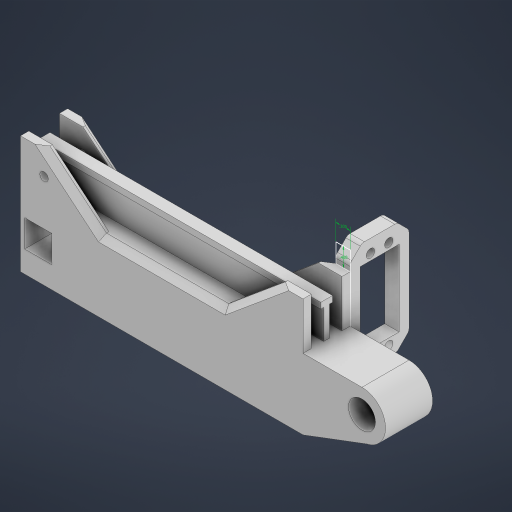
# Autodesk Inventor part: Drone_Launcher_Base2
Saved by Autodesk Inventor 2023 (Build 270158000, 158)
## iProperties
Created: 2024-02-18
Part Number: Drone_Launcher_Base2
Material: Generic
Document SubType Name: Modeling
Designer: kelle
Density: 1 g/cm^3
Appearance: Default
Author: kelle
Autodesk Inventor part; units mm, degrees
ref_plane "YZ Plane" through (0, 0, 0) normal (1, 0, 0) x (0, 1, 0)
ref_plane "XZ Plane" through (0, 0, 0) normal (0, 1, 0) x (-1, 0, 0)
ref_plane "XY Plane" through (0, 0, 0) normal (0, 0, 1) x (1, 0, 0)
sketch "Sketch1" plane through (0, 0, 0) normal (0, 0, 1) x (1, 0, 0)
  line L0 (76.2, -19.05) -> (-76.2, -19.05)
  line L1 (-76.2, -19.05) -> (-76.2, 19.05)
  line L2 (-76.2, 19.05) -> (76.2, 19.05)
  line L3 (76.2, 19.05) -> (76.2, -19.05)
  line L4 (76.2, -19.05) -> (-76.2, 19.05) construction
  line L5 (-76.2, -19.05) -> (76.2, 19.05) construction
  circle A0 centre (107.95, 6.35) radius 7.25
  circle A1 centre (107.95, 6.35) radius 12.7
  line L6 (76.2, 19.05) -> (107.95, 19.05)
  line L7 (-76.2, 19.05) -> (-57.1396, 19.05)
  line L8 (-57.1396, 19.05) -> (-57.1396, -9.525)
  line L9 (-57.1396, -9.525) -> (-76.2, -9.525)
  line L10 (-76.2, -9.525) -> (-76.2, 19.05)
  line L11 (-57.1396, -9.525) -> (-47.6146, 0)
  line L12 (-57.1396, -9.525) -> (-43.6692, -9.525) construction
  line L13 (-47.6146, 0) -> (0, 0)
  line L14 (-59.3621, -7.3025) -> (-73.9671, -7.3025)
  line L15 (-73.9671, -7.3025) -> (-73.9671, 7.3025)
  line L16 (-73.9671, 7.3025) -> (-59.3621, 7.3025)
  line L17 (-59.3621, 7.3025) -> (-59.3621, -7.3025)
  line L18 (-59.3621, -7.3025) -> (-73.9671, 7.3025) construction
  line L19 (-73.9671, -7.3025) -> (-59.3621, 7.3025) construction
  line L20 (-76.2, 19.05) -> (-76.2, 44.45)
  line L21 (-76.2, 44.45) -> (-63.5, 44.45)
  line L22 (76.2, 19.05) -> (76.2, 44.45)
  line L23 (76.2, 44.45) -> (63.5, 44.45)
  line L24 (-33.0096, 19.05) -> (-33.0096, -19.05) construction
  line L25 (0, 19.05) -> (0, -19.05) construction
  line L26 (33.0096, 19.05) -> (33.0096, -19.05) construction
  line L27 (-63.5, 44.45) -> (-33.0096, 19.05)
  line L28 (33.0096, 19.05) -> (63.5, 44.45)
  circle A2 centre (-63.5, 31.75) radius 2.25
  line L29 (76.2, 19.05) -> (107.95, 19.05)
  line L30 (76.2, -19.05) -> (114.0984, -4.7625)
  point P0 (107.95, -6.35)
  point P1 (-66.6646, 0)
  point P2 (110.6679, -6.0558)
  dimension "d0" = 152.4
  dimension "d1" = 38.1
  dimension "d4" = 14.5
  dimension "d5" = 25.4
  dimension "d7" = 12.7
  dimension "d8" = 28.575
  dimension "d9" = 45
  dimension "d10" = 19.0604
  dimension "d12" = 14.605
  dimension "d13" = 14.605
  dimension "d14" = 2.2225
  dimension "d15" = 2.2225
  dimension "d16" = 25.4
  dimension "d17" = 12.7
  dimension "d18" = 25.4
  dimension "d19" = 12.7
  dimension "d20" = 33.0096
  dimension "d21" = 4.5
  dimension "d22" = 12.7
  dimension "d23" = 12.7
  dimension "d88" = 31.75
  constraints: 62 end point, 7 perpendicular, 6 midpoint, 6 parallel, 5 horizontal, 4 point on line, 3 centre point, 3 point on circle, 2 symmetric about line, 1 coincident, 1 equal length
  measures "d0" distance of L1.end L2.end
  measures "d1" distance of L0.end L1.end
  measures "d4" diameter of A0
  measures "d5" diameter of A1
  measures "d7" distance from line of L2 A1.centre
  measures "d8" distance of L7.end L8.end
  measures "d9" angle of L12 L11
  measures "d10" distance between parallel lines of L1 L8
  measures "d12" distance of L15.end L16.end
  measures "d13" distance of L14.end L15.end
  measures "d14" distance between parallel lines of L8 L17
  measures "d15" distance between parallel lines of L9 L14
  measures "d16" distance of L1.end L20.end
  measures "d17" distance of L20.end L21.end
  measures "d18" distance of L2.end L22.end
  measures "d19" distance of L22.end L23.end
  measures "d20" distance between parallel lines of L25 L24
  measures "d21" diameter of A2
  measures "d22" distance from line of L21 A2.centre
  measures "d23" distance from line of L20 A2.centre
  measures "d88" distance from line of L3 A0.centre
extrude "Extrusion1" add sketch "Sketch1" along normal blind 25.4
sketch "Sketch2" plane through (-76.2, -9.525, 0) normal (-1, 0, 0) x (0, 0, 1)
  line L0 (0, 53.975) -> (0, -9.525) projected
  line L1 (25.4, 53.975) -> (25.4, -9.525) projected
  line L2 (0, 53.975) -> (25.4, 53.975) projected
  line L3 (0, 28.575) -> (25.4, 28.575) projected
  line L4 (0, 28.575) -> (25.4, 28.575) construction
  line L5 (12.7, 28.575) -> (12.7, 53.975) construction
  line L6 (0, 53.975) -> (25.4, 53.975) construction
  line L7 (0, 28.575) -> (25.4, 53.975) construction
  line L8 (20.955, 28.575) -> (4.445, 28.575) construction
  line L9 (4.445, 28.575) -> (4.445, 53.975)
  line L10 (4.445, 53.975) -> (20.955, 53.975) construction
  line L11 (20.955, 53.975) -> (20.955, 28.575)
  line L12 (20.955, 28.575) -> (4.445, 53.975) construction
  line L13 (4.445, 28.575) -> (20.955, 53.975) construction
  circle A0 centre (4.445, 22.225) radius 2.85
  circle A1 centre (20.955, 22.225) radius 2.85
  line L14 (0, -9.525) -> (25.4, -9.525) projected
  point P0 (0, 9.525)
  point P1 (12.7, 41.275)
  dimension "d26" = 16.51
  dimension "d39" = 5.7
  dimension "d40" = 5.7
  dimension "d43" = 6.35
  dimension "d44" = 6.35
  constraints: 16 end point, 5 midpoint, 2 centre point, 2 parallel, 1 horizontal, 1 perpendicular, 1 point on line
  measures "d26" distance of L9.end L10.end
  measures "d39" diameter of A0
  measures "d40" diameter of A1
  measures "d43" distance from line of L3 A1.centre
  measures "d44" distance from line of L3 A0.centre
extrude "Extrusion2" cut sketch "Sketch2" against normal up to surface (139.7 mm away) contours L2 L11 L3 L9
sketch "Sketch3" plane through (-33.0096, 19.05, 0) normal (0, 1, 0) x (1, 0, 0)
  line L0 (33.0096, 0) -> (33.0096, -24.4883) construction
  line L1 (-43.1904, 0) -> (-43.1904, -25.4) construction
  line L2 (-43.1904, -12.7) -> (96.5096, -12.7) construction
  line L3 (96.5096, -4.445) -> (96.5096, -20.955) construction
  line L4 (-43.1904, -14.2875) -> (98.7956, -14.2875)
  line L5 (98.7956, -14.2875) -> (98.7956, -11.1125)
  line L6 (98.7956, -11.1125) -> (-43.1904, -11.1125)
  line L7 (-43.1904, -11.1125) -> (-43.1904, -14.2875)
  line L8 (-43.1904, -14.2875) -> (98.7956, -11.1125) construction
  line L9 (98.7956, -14.2875) -> (-43.1904, -11.1125) construction
  point P0 (27.8026, -12.7)
  point P1 (-43.1904, -12.7)
  dimension "d29" = 141.986
  dimension "d30" = 3.175
  dimension "d31" = 0
  constraints: 16 end point, 5 midpoint, 2 parallel, 1 horizontal, 1 perpendicular, 1 point on line, 1 vertical
  measures "d29" distance of L6.end L5.end
  measures "d30" distance of L5.end L4.end
  measures "d31" distance from line of L1 point (-43.19, -12.7)
extrude "Extrusion3" add sketch "Sketch3" along normal blind 19.05
sketch "Sketch4" plane through (-76.2, -9.525, 0) normal (-1, 0, 0) x (0, 0, 1)
  line L0 (11.1125, 47.625) -> (14.2875, 47.625) construction
  line L1 (12.7, 47.625) -> (12.7, 0) construction
  line L2 (0, 0) -> (25.4, 0) construction
  line L3 (15.875, 44.45) -> (9.525, 44.45)
  line L4 (9.525, 44.45) -> (9.525, 47.625)
  line L5 (9.525, 47.625) -> (15.875, 47.625)
  line L6 (15.875, 47.625) -> (15.875, 44.45)
  line L7 (15.875, 44.45) -> (9.525, 47.625) construction
  line L8 (9.525, 44.45) -> (15.875, 47.625) construction
  point P0 (0, 9.525)
  point P1 (12.7, 46.0375)
  dimension "d34" = 6.35
  dimension "d35" = 3.175
  dimension "d36" = 0
  constraints: 14 end point, 4 midpoint, 2 parallel, 1 horizontal, 1 perpendicular, 1 point on line
  measures "d34" distance of L4.end L5.end
  measures "d35" distance of L3.end L4.end
  measures "d36" distance between parallel lines of L0 L5
extrude "Extrusion4" add sketch "Sketch4" against normal up to surface (139.7 mm away)
extrude "Extrusion5" cut sketch "Sketch2" against normal blind 9 contours A0 | A1
chamfer "Chamfer1" distance 3.175 angle 45 6 edges at (0, 19.05, 25.4) (48.2548, 31.75, 25.4) (-48.2548, 31.75, 25.4) (48.2548, 31.75, 0) (0, 19.05, 0) (-48.2548, 31.75, 0)
chamfer "Chamfer2" [suppressed]
sketch "Sketch5" plane through (63.5, 19.05, 20.955) normal (-1, 0, 0) x (0, 0, 1)
  line L0 (-11.43, 19.05) -> (-5.08, 19.05) projected
  line L1 (-5.08, 19.05) -> (-5.08, 15.875) projected
  line L2 (-5.08, 15.875) -> (-6.6675, 15.875) projected
  line L3 (-6.6675, 15.875) -> (-6.6675, 0) projected
  line L4 (0, 0) -> (-6.6675, 0) projected
  line L5 (0, 25.4) -> (0, 0) projected
  line L6 (-16.51, 25.4) -> (0, 25.4) projected
  line L7 (-16.51, 0) -> (-16.51, 25.4) projected
  line L8 (-9.8425, 0) -> (-16.51, 0) projected
  line L9 (-9.8425, 0) -> (-9.8425, 15.875) projected
  line L10 (-9.8425, 15.875) -> (-11.43, 15.875) projected
  line L11 (-11.43, 15.875) -> (-11.43, 19.05) projected
  point P0 (-20.955, -19.05)
extrude "Extrusion6" cut sketch "Sketch5" against normal through all
sketch "Sketch6" plane through (0, 0, 0) normal (0, 0, -1) x (-1, 0, 0)
  line L0 (-76.2, 44.45) -> (-68.4605, 44.45) projected
  line L1 (-76.2, 44.45) -> (-76.2, -5.4429)
  line L2 (44.45, 3.175) -> (-88.9, -6.35) projected
  line L3 (-68.4605, 44.45) -> (-34.1588, 15.875) construction
  line L4 (-68.4605, 44.45) -> (-68.4605, -5.4429)
  line L5 (-76.2, 44.45) -> (-68.453, 44.45)
  line L6 (-68.453, 44.45) -> (-68.453, 54.61)
  line L7 (-68.453, 54.61) -> (-76.2, 54.61)
  line L8 (-76.2, 54.61) -> (-76.2, 44.45)
  point P0 (0, 0)
  point P1 (-68.4605, -4.89)
  point P2 (-72.3265, 54.61)
  point P3 (-68.4605, 44.45)
  dimension "d57" = 7.747
  dimension "d58" = 10.16
  constraints: 12 end point, 2 parallel, 2 vertical, 1 horizontal, 1 midpoint, 1 perpendicular, 1 point on line
  measures "d57" distance of L7.end L6.end
  measures "d58" distance from line of L0 point (-72.326, 54.61)
extrude "Extrusion7" add sketch "Sketch6" along normal blind 31.75
chamfer "Chamfer3" distance 6.35 angle 45 3 edges at (72.3265, 54.61, -31.75) (72.3303, -5.1664, -31.75) (72.3265, 54.61, 0)
fillet "Fillet1" radius 3.175 5 edges at (72.3303, 1.1997, -31.75) (72.3265, 48.26, -31.75) (72.3265, 54.61, -25.4) (72.3265, 54.61, -6.35) (72.3265, 48.26, 0)
sketch "Sketch9" plane through (0, 0, 0) normal (0, 0, -1) x (-1, 0, 0)
  line L0 (44.45, 3.175) -> (-88.9, -6.35) projected
  line L1 (58.4547, -6.35) -> (57.1396, -9.525) projected
  line L2 (-88.9, -6.35) -> (57.1396, -9.525)
  line L3 (-68.4605, 44.45) -> (-68.4605, -4.89) projected
  line L4 (76.2, 44.45) -> (76.2, -19.05) projected
  line L5 (68.4605, 44.45) -> (76.2, 44.45) projected
  line L6 (34.1588, 15.875) -> (68.4605, 44.45) projected
  line L7 (-34.1588, 15.875) -> (34.1588, 15.875) projected
  line L8 (-68.4605, 44.45) -> (-34.1588, 15.875) projected
  line L9 (-68.4605, -4.89) -> (-76.2, -5.4429) projected
  line L10 (76.2, -19.05) -> (-76.2, -19.05) projected
  line L11 (-76.2, -5.4429) -> (-76.2, 19.05) projected
  line L12 (-107.95, 19.05) -> (-76.2, 19.05) projected
  arc A0 (-107.95, 19.05) -> (-110.6679, -6.0558) centre (-107.95, 6.35) ccw projected
  line L13 (-76.2, -19.05) -> (-110.6679, -6.0558) projected
  point P0 (0, 0)
  constraints: 2 end point
extrude "Extrusion11" [suppressed]
sketch "Sketch10" plane through (76.2, -5.4429, 0) normal (1, 0, 0) x (0, 0, -1)
  circle A0 centre (10.925, 4.3029) radius 2.25 projected
  circle A1 centre (20.825, 52.3029) radius 2.25 projected
  circle A2 centre (20.825, 4.3029) radius 2.25 projected
  circle A3 centre (10.925, 52.3029) radius 2.25 projected
  arc A4 (0.9299, 54.6328) -> (0, 52.3877) centre (3.175, 52.3877) ccw projected
  line L0 (0, 52.3877) -> (0, 49.8929) projected
  line L1 (0, 49.8929) -> (-4.445, 49.8929) projected
  line L2 (-4.445, 49.8929) -> (-4.445, 24.4929) projected
  line L3 (0, 24.4929) -> (-4.445, 24.4929) projected
  line L4 (0, 0) -> (0, 24.4929) projected
  line L5 (0, 0) -> (24.0849, 0) projected
  ellipse E0 centre (24.0849, 3.1831) end of major axis (24.0849, 0) minor radius 3.175 (24.0849, 0) -> (26.3299, 0.9323) ccw projected
  line L6 (27.7824, 2.3885) -> (26.3299, 0.9323) projected
  ellipse E1 centre (25.526, 4.6279) end of major axis (28.709, 4.6279) minor radius 3.175 (27.7824, 2.3885) -> (25.526, 7.8029) ccw projected
  line L7 (25.526, 7.8029) -> (4.625, 7.8029) projected
  line L8 (4.625, 7.8029) -> (4.625, 48.8029) projected
  line L9 (4.625, 48.8029) -> (28.575, 48.8029) projected
  arc A5 (28.575, 48.8029) -> (31.75, 51.9779) centre (28.575, 51.9779) ccw projected
  line L10 (31.75, 52.3877) -> (31.75, 51.9779) projected
  arc A6 (31.75, 52.3877) -> (30.8201, 54.6328) centre (28.575, 52.3877) ccw projected
  line L11 (26.3299, 59.1229) -> (30.8201, 54.6328) projected
  arc A7 (26.3299, 59.1229) -> (24.0849, 60.0529) centre (24.0849, 56.8779) ccw projected
  line L12 (7.6651, 60.0529) -> (24.0849, 60.0529) projected
  arc A8 (7.6651, 60.0529) -> (5.4201, 59.1229) centre (7.6651, 56.8779) ccw projected
  line L13 (0.9299, 54.6328) -> (5.4201, 59.1229) projected
  line L14 (-4.445, 49.8929) -> (-4.445, 24.4929) projected
  line L15 (-4.445, 49.8929) -> (0.2417, 53.6027)
  point P0 (0, 5.4429)
  constraints: 2 end point, 1 point on circle, 2 other
extrude "Extrusion12" [suppressed]
sketch "Sketch11" plane through (76.2, 19.05, 4.445) normal (1, 0, 0) x (0, 0, -1)
  line L0 (12.1101, 35.56) -> (28.5299, 35.56) construction
  line L1 (20.32, 35.56) -> (20.32, -23.94) construction
  line L2 (4.445, -23.94) -> (29.845, -23.94) construction
  line L3 (36.195, -16.2554) -> (36.195, 25.4) construction
  line L4 (36.195, 4.5723) -> (4.445, 4.5723) construction
  line L5 (4.445, 25.4) -> (4.445, -3.175) construction
  line L6 (30.82, -15.9277) -> (9.82, -15.9277)
  line L7 (9.82, -15.9277) -> (9.82, 25.0723)
  line L8 (9.82, 25.0723) -> (30.82, 25.0723)
  line L9 (30.82, 25.0723) -> (30.82, -15.9277)
  line L10 (30.82, -15.9277) -> (9.82, 25.0723) construction
  line L11 (9.82, -15.9277) -> (30.82, 25.0723) construction
  circle A0 centre (25.27, 28.5723) radius 2.25
  circle A1 centre (25.27, -19.4277) radius 2.25
  circle A2 centre (15.37, 28.5723) radius 2.25
  circle A3 centre (15.37, -19.4277) radius 2.25
  point P0 (4.445, -19.05)
  point P1 (20.32, 4.5723)
  dimension "d89" = 21
  dimension "d90" = 41
  dimension "d91" = 24
  dimension "d92" = 4.5
  dimension "d93" = 4.95
  dimension "d96" = 48
  dimension "d99" = 9.9
  constraints: 16 end point, 5 midpoint, 4 centre point, 3 horizontal, 2 parallel, 2 point on line, 2 vertical, 1 perpendicular, 6 other
  measures "d89" distance of L7.end L8.end
  measures "d90" distance of L6.end L7.end
  measures "d91" distance from line of L4 A0.centre
  measures "d92" diameter of A0
  measures "d93" distance from line of L1 A0.centre
  measures "d96" distance of A0.centre A1.centre
  measures "d99" distance of A0.centre A2.centre
extrude "Extrusion13" cut sketch "Sketch11" against normal through all
body "Solid1"
